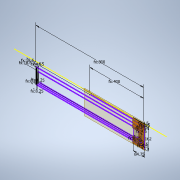
# Autodesk Inventor part: primary_coil_0R2_test_cut
Saved by Autodesk Inventor 2021 (Build 250183000, 183)
## iProperties
Created: 2021-01-20
Part Number: primary_coil_0R2_test_cut
Material: Generic
Document SubType Name: Modeling
Designer: phamv
Density: 1 g/cm^3
Appearance: Default
Author: phamv
Autodesk Inventor part; units mm, degrees
ref_plane "YZ Plane" through (0, 0, 0) normal (1, 0, 0) x (0, 1, 0)
sketch "Sketch1" plane through (0, 0, 0) normal (0, 0, 1) x (1, 0, 0)
  line L0 (6.5, -9.3) -> (385, -9.3)
  line L1 (400, -24.3) -> (400, -135)
  line L2 (385, -150) -> (-400, -150)
  line L3 (-400, -150) -> (-400, -32.4)
  line L4 (6.5, -9.3) -> (6.5, -13.8)
  line L5 (6.5, -13.8) -> (380.5, -13.8)
  line L6 (395.5, -28.8) -> (395.5, -130.5)
  line L7 (380.5, -145.5) -> (-395.5, -145.5)
  line L8 (-400, -32.4) -> (375.5, -32.4)
  line L9 (390.5, -47.4) -> (390.5, -122.25)
  line L10 (375.5, -137.25) -> (-387.25, -137.25)
  line L11 (-395.5, -145.5) -> (-395.5, -36.9)
  line L12 (-395.5, -36.9) -> (371, -36.9)
  line L13 (386, -51.9) -> (386, -117.75)
  line L14 (371, -132.75) -> (-382.75, -132.75)
  line L15 (-382.75, -132.75) -> (-382.75, -60)
  line L16 (-387.25, -137.25) -> (-387.25, -55.5)
  line L17 (-387.25, -55.5) -> (366, -55.5)
  line L18 (381, -70.5) -> (381, -109.5)
  line L19 (-382.75, -60) -> (361.5, -60)
  line L20 (376.5, -75) -> (376.5, -105)
  line L21 (361.5, -120) -> (-374.5, -120)
  line L22 (366, -124.5) -> (-374.5, -124.5)
  line L23 (-374.5, -124.5) -> (-374.5, -120)
  arc A0 (400, -24.3) -> (385, -9.3) centre (385, -24.3) ccw
  arc A1 (395.5, -28.8) -> (380.5, -13.8) centre (380.5, -28.8) ccw
  arc A2 (390.5, -47.4) -> (375.5, -32.4) centre (375.5, -47.4) ccw
  arc A3 (386, -51.9) -> (371, -36.9) centre (371, -51.9) ccw
  arc A4 (381, -70.5) -> (366, -55.5) centre (366, -70.5) ccw
  arc A5 (376.5, -75) -> (361.5, -60) centre (361.5, -75) ccw
  arc A6 (361.5, -120) -> (376.5, -105) centre (361.5, -105) ccw
  arc A7 (366, -124.5) -> (381, -109.5) centre (366, -109.5) ccw
  arc A8 (371, -132.75) -> (386, -117.75) centre (371, -117.75) ccw
  arc A9 (375.5, -137.25) -> (390.5, -122.25) centre (375.5, -122.25) ccw
  arc A10 (380.5, -145.5) -> (395.5, -130.5) centre (380.5, -130.5) ccw
  arc A11 (385, -150) -> (400, -135) centre (385, -135) ccw
  line L24 (322.4983, 0) -> (322.4983, -162)
  line L25 (322.4983, -162) -> (407.2483, -162)
  line L26 (407.2483, -162) -> (407.2483, 0)
  line L27 (407.2483, 0) -> (322.4983, 0)
  line L28 (-561.4497, 0) -> (568.6979, 0) projected
  line L29 (322.4983, -123.614) -> (322.4983, -76.5697)
  line L30 (322.4983, -65.8872) -> (366.8197, -65.8872)
  line L31 (366.8197, -65.8872) -> (366.8197, -114.4349)
  line L32 (366.8197, -114.4349) -> (322.4983, -114.4349)
  point P0 (0, 0)
  point P1 (400, -9.3)
  point P2 (400, -150)
  point P3 (395.5, -13.8)
  point P4 (395.5, -145.5)
  point P5 (390.5, -32.4)
  point P6 (390.5, -137.25)
  point P7 (386, -36.9)
  point P8 (386, -132.75)
  point P9 (381, -55.5)
  point P10 (381, -124.5)
  point P11 (376.5, -60)
  point P12 (376.5, -120)
  point P13 (0, 0)
  point P14 (322.4983, -60)
  point P15 (322.4983, -120)
  point P16 (322.4983, -36.9)
  point P17 (322.4983, -55.5)
  point P18 (322.4983, -124.5)
  point P19 (322.4983, -132.75)
  point P20 (322.4983, -13.8)
  point P21 (322.4983, -32.4)
  point P22 (322.4983, -137.25)
  point P23 (322.4983, -145.5)
  point P24 (322.4983, -150)
  point P25 (322.4983, -9.3)
  dimension "d1" = 4.5
  dimension "d2" = 4.5
  dimension "d3" = 4.5
  dimension "d5" = 800
  dimension "d6" = 400
  dimension "d7" = 4.5
  dimension "d8" = 4.5
  dimension "d9" = 5
  dimension "d10" = 4.5
  dimension "d11" = 18.6
  dimension "d12" = 4.5
  dimension "d13" = 8.25
  dimension "d14" = 4.5
  dimension "d15" = 4.5
  dimension "d16" = 4.5
  dimension "d17" = 5
  dimension "d19" = 18.6
  dimension "d20" = 8.25
  dimension "d89" = 8.25
  dimension "d90" = 8.25
  dimension "d91" = 15
  dimension "d104" = 84.75
  dimension "d106" = 162
  constraints: 64 end point, 27 point on line, 24 point on circle, 24 tangent, 18 perpendicular, 12 centre point, 11 equal radius, 5 horizontal, 3 parallel, 3 vertical, 1 coincident, 1 collinear
  measures "d1" distance between parallel lines of L5 L0
  measures "d2" distance between parallel lines of L6 L1
  measures "d3" distance between parallel lines of L2 L7
  measures "d5" distance between parallel lines of L3 L1
  measures "d6" distance from line of point (0, 0) L1
  measures "d7" distance between parallel lines of L3 L11
  measures "d8" distance between parallel lines of L13 L9
  measures "d9" distance between parallel lines of L9 L6
  measures "d10" distance between parallel lines of L8 L12
  measures "d11" distance between parallel lines of L8 L5
  measures "d12" distance between parallel lines of L10 L14
  measures "d13" distance between parallel lines of L7 L10
  measures "d14" distance between parallel lines of L16 L15
  measures "d15" distance between parallel lines of L17 L19
  measures "d16" distance between parallel lines of L20 L18
  measures "d17" distance between parallel lines of L18 L13
  measures "d19" distance between parallel lines of L17 L12
  measures "d20" distance between parallel lines of L11 L16
  measures "d89" distance between parallel lines of L14 L22
  measures "d90" distance between parallel lines of L15 L23
  measures "d91" radius of A0
  measures "d104" distance between parallel lines of L26 L24
  measures "d106" distance between parallel lines of L25 L27
extrude "Extrusion1" add sketch "Sketch1" along normal blind 4.5 contours L24 L27 L26 L25 L2 A11 L1 A0 L0 | L5 A1 L6 A10 L7 L24 L10 A9 L9 A2 L8 | L12 A3 L13 A8 L14 L24 L22 A7 L18 A4 L17 | L19 A5 L20 A6 L21 L24 L32 L31 L30
extrude "Extrusion7" add sketch "Sketch1" against normal blind 0.45 contours L24 L27 L26 L25 L2 A11 L1 A0 L0 | L0 A0 L1 A11 L2 L24 L7 A10 L6 A1 L5 | L5 A1 L6 A10 L7 L24 L10 A9 L9 A2 L8 | L8 A2 L9 A9 L10 L24 L14 A8 L13 A3 L12 | L12 A3 L13 A8 L14 L24 L22 A7 L18 A4 L17 | L17 A4 L18 A7 L22 L24 L21 A6 L20 A5 L19 | L19 A5 L20 A6 L21 L24 L32 L31 L30 | L30 L31 L32 L24
equation "\"d1\" = wire_diameter"
equation "\"d2\" = wire_diameter"
equation "\"d3\" = wire_diameter"
equation "\"d5\" = track_length"
equation "\"d6\" = 0.5 * track_length"
equation "\"d7\" = wire_diameter"
equation "\"d8\" = wire_diameter"
equation "\"d10\" = wire_diameter"
equation "\"d11\" = distance_between_wires"
equation "\"d12\" = wire_diameter"
equation "\"d13\" = distance_between_wires_edge"
equation "\"d14\" = wire_diameter"
equation "\"d15\" = wire_diameter"
equation "\"d16\" = wire_diameter"
equation "\"d19\" = distance_between_wires"
equation "\"d20\" = distance_between_wires_edge"
equation "\"d22\" = wire_diameter"
equation "\"track_length\" = 800"
equation "\"wire_diameter\" = 4.5"
equation "\"distance_between_wires\" = -1.2 * wire_diameter + 0.2 * parameter_6"
equation "\"distance_between_wires_edge\" = 8.25"
equation "\"bend_radius\" = 15"
equation "\"parameter_6\" = 120"
body "Solid1"
